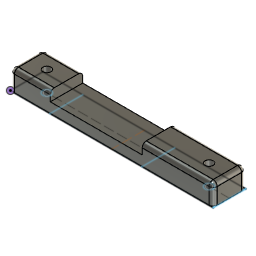
droy-top v2 (Autodesk Fusion 360 design; units mm, degrees)
Autodesk Fusion 360 part; units mm, degrees
sketch "Sketch1" plane through (0, 0, 0) normal (0, 0, 1) x (1, 0, 0)
  line L0 (0, 0) -> (100, 0)
  line L1 (100, 0) -> (100, 16)
  line L2 (100, 16) -> (0, 16)
  line L3 (0, 16) -> (0, 0)
  line L4 (0, 8) -> (100, 8) construction
  line L5 (50, 16) -> (50, 0) construction
  circle A0 centre (10, 8) radius 2
  circle A1 centre (90, 8) radius 2
  line L6 (19.6419, 16) -> (19.6419, 0)
  line L7 (65, 16) -> (65, 0)
  dimension "d1" = 16
  dimension "d2" = 4
  dimension "d3" = 4
  dimension "d4" = 40
  dimension "d5" = 40
  dimension "d22" = 35
  constraint horizontal L0
  constraint vertical L1
  constraint horizontal L2
  constraint vertical L3
  constraint coincident L0.start L3.end
  constraint midpoint L3 L4.start
  constraint midpoint L1 L4.end
  constraint midpoint L2 L5.start
  constraint midpoint L0 L5.end
  constraint coincident L4 A0.centre
  constraint coincident L4 A1.centre
  constraint coincident L2 L6.start
  constraint perpendicular L2 L6
  constraint coincident L0 L6.end
  constraint coincident L2 L7.start
  constraint perpendicular L2 L7
  constraint coincident L0 L7.end
  measures "d1" distance of L0.start L2.end
  measures "d2" diameter of A0
  measures "d3" diameter of A1
  measures "d4" distance of L5 A0.centre
  measures "d5" distance of L5 A1.centre
  measures "d22" distance of L1 L7
extrude "Extrude1" add sketch "Sketch1" along normal blind 10 contours L0 L2 L3 L6 | L0 L1 L2 L7 makes body 1 at (2.6667, 8, 0) makes body 2 at (72.6667, 8, 0)
extrude "Extrude2" add sketch "Sketch1" along normal blind 5 contours L0 L2 L6 L7 bodies 1 2
fillet "Fillet1" radius 2 1 edges at (0, 8, 10) on bodies 1
fillet "Fillet2" radius 2 1 edges at (100, 8, 10) on bodies 1
fillet "Fillet3" radius 2 3 edges at (0, 16, 4) (0.5858, 16, 9.4142) (10.821, 16, 10) on bodies 1
fillet "Fillet4" radius 2 3 edges at (100, 16, 4) (99.4142, 16, 9.4142) (81.5, 16, 10) on bodies 1
fillet "Fillet5" radius 2 3 edges at (0, 0, 4) (0.5858, 0, 9.4142) (10.821, 0, 10) on bodies 1
fillet "Fillet6" radius 2 3 edges at (81.5, 0, 10) (99.4142, 0, 9.4142) (100, 0, 4) on bodies 1
